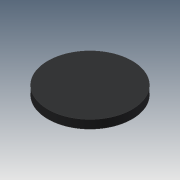
# Autodesk Inventor part: FLUGGER SORBOTHANE BUMPER
Saved by Autodesk Inventor 2020.3 (Build 243373000, 373)
## iProperties
Created: 2023-03-28
Part Number: FLUGGER SORBOTHANE BUMPER
Material: RUBBER, EPDM
Catalog Web Link: https://www.janelia.org/
Vendor: HHMI: JRC - jET
Document SubType Name: Modeling
Designer: arnoldj
Density: 0.86 g/cm^3
Appearance: Rubber (Black)
RuleStatus: InUse
AfterDocSave0: file://Part Number Cleaner
Title: Standard
Author: arnoldj
Revision Number: 0
DESIGN DEPARTMENT: HHMI: JRC - jET
ALTERED ITEM PART NUMBER: N/A
ALTERED ITEM VENDOR: N/A
ALTERED ITEM DESCRIPTION: N/A
Autodesk Inventor part; units mm, degrees
ref_plane "YZ Plane" through (0, 0, 0) normal (1, 0, 0) x (0, 1, 0)
ref_plane "XZ Plane" through (0, 0, 0) normal (0, 1, 0) x (-1, 0, 0)
ref_plane "XY Plane" through (0, 0, 0) normal (0, 0, 1) x (1, 0, 0)
sketch "Sketch1" plane through (0, 0, 0) normal (0, 1, 0) x (-1, 0, 0)
  line L0 (0, -44.45) -> (0, 44.45) projected
  line L1 (-44.45, 0) -> (44.45, 0) projected
  circle A0 centre (0, 0) radius 31.75
  dimension "d0" = 63.5
  constraints: 1 centre point, 1 coincident
  measures "d0" diameter of A0
extrude "Extrusion1" add sketch "Sketch1" against normal blind 6.35
body "Solid1"
